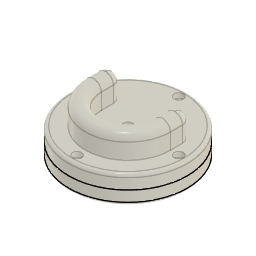
Spool Rod Holder (Autodesk Fusion 360 design; units mm, degrees)
Autodesk Fusion 360 part; units mm, degrees
sketch "Sketch1" plane through (0, 0, 0) normal (0, 0, 1) x (1, 0, 0) in component "Internal Rod Holder"
  circle A0 centre (0, 0) radius 16.875
  circle A1 centre (0, 0) radius 26.875
  line L0 (0, 16.875) -> (30, 16.875) construction
  line L1 (0, 16.875) -> (-30, 16.875) construction
  line L2 (-21.5932, 16) -> (-11.5932, 16)
  line L3 (-11.5932, 16) -> (-11.5932, 16.875)
  line L4 (-11.5932, 16.875) -> (-21.5932, 16.875)
  line L5 (-21.5932, 16.875) -> (-21.5932, 16)
  line L6 (5.3634, 16) -> (15.3634, 16)
  line L7 (15.3634, 16) -> (15.3634, 16.875)
  line L8 (15.3634, 16.875) -> (5.3634, 16.875)
  line L9 (5.3634, 16.875) -> (5.3634, 16)
  circle A2 centre (0, 0) radius 37.5
  line L10 (-33.9153, 16) -> (33.9153, 16)
  line L11 (-33.9153, 16) -> (-21.5932, 16)
  line L12 (15.3634, 16) -> (33.9153, 16)
  line L13 (0.0001, -26.875) -> (0.0001, -37.5)
  line L14 (0.0001, 26.875) -> (0.0001, 37.5)
  line L15 (-26.875, 0) -> (-37.5, 0)
  line L16 (26.875, 0) -> (37.5, 0)
  point P0 (-32, 16)
  point P1 (0.0001, 32.1875)
  point P2 (24.6393, 16)
  point P3 (-32.1875, 0)
  point P4 (32.1875, 0)
  point P5 (0.0001, -32.1875)
  dimension "d2" = 33.75
  dimension "d3" = 53.75
  dimension "d4" = 10
  dimension "d5" = 10
  dimension "d6" = 75
  dimension "d28" = 10.625
  constraint coincident A0.centre A1.centre
  constraint concentric A0 A1
  constraint coincident A0 L0.start
  constraint tangent A0 L0
  constraint horizontal L0
  constraint tangent A0 L1
  constraint horizontal L2
  constraint vertical L3
  constraint horizontal L4
  constraint vertical L5
  constraint coincident A1 L2.start
  constraint horizontal L6
  constraint vertical L7
  constraint horizontal L8
  constraint vertical L9
  constraint coincident A0 L6.start
  constraint concentric A1 A2
  constraint coincident A2 L10.start
  constraint coincident A2 L10.end
  constraint parallel L6 L10
  constraint coincident L10 P0
  constraint perpendicular L5 L11
  constraint perpendicular L7 L12
  constraint coincident A1 L13.start
  constraint coincident A2 L13.end
  constraint perpendicular L0 L13
  constraint coincident A1 L14.start
  constraint coincident A2 L14.end
  constraint parallel L13 L14
  constraint midpoint L14 P1
  constraint midpoint L12 P2
  constraint coincident A1 L15.start
  constraint coincident A2 L15.end
  constraint horizontal L15
  constraint coincident A1 L16.start
  constraint coincident A2 L16.end
  constraint parallel L15 L16
  constraint midpoint L15 P3
  constraint midpoint L16 P4
  constraint horizontal P3 P4
  constraint midpoint L13 P5
  measures "d2" diameter of A0
  measures "d3" diameter of A1
  measures "d4" distance of L2.start L2.end
  measures "d5" distance of L6.start L6.end
  measures "d6" diameter of A2
  measures "d28" distance of A1 A2
cylinder "CylinderPrimitive1" add diameter 75 height 8.75 placed x (1, 0, 0) y (0, 1, 0) z (0, 0, 1) at (0, 0, 0) makes body 1 in component "Internal Rod Holder"
cylinder "CylinderPrimitive2" add diameter 53.75 height 15 placed x (1, 0, 0) y (0, 1, 0) z (0, 0, 1) at (0, 0, 8.75) bodies 1 in component "Internal Rod Holder"
box "BoxPrimitive1" cut length 27.0154 width 53.75 height -15 placed x (0, 1, 0) y (-1, 0, 0) z (0, 0, 1) at (26.875, 0, 23.75) bodies 1 in component "Internal Rod Holder"
cylinder "CylinderPrimitive3" cut diameter 33.75 height 15 placed x (1, 0, 0) y (0, 1, 0) z (0, 0, 1) at (0, 0, 8.75) bodies 1 in component "Internal Rod Holder"
box "BoxPrimitive2" add length 12.656 width 10 height 15 placed x (0, 1, 0) y (-1, 0, 0) z (0, 0, 1) at (-16.875, 0, 8.75) bodies 1 in component "Internal Rod Holder"
box "BoxPrimitive3" add length 12.656 width 10 height 15 placed x (0, 1, 0) y (-1, 0, 0) z (0, 0, 1) at (26.875, 0, 8.75) bodies 1 in component "Internal Rod Holder"
sketch "Sketch8" plane through (0, 0, 8.75) normal (0, 0, 1) x (-1, 0, 0) in component "Internal Rod Holder"
  line L0 (-16.875, 0) -> (-16.875, -12.656)
  line L1 (-16.875, -12.656) -> (-26.875, -12.656)
  line L2 (-26.875, -12.656) -> (-26.875, 0)
  arc A0 (26.875, 0) -> (-26.875, 0) centre (0, 0) ccw
  line L3 (26.875, 0) -> (26.875, -12.656)
  line L4 (26.875, -12.656) -> (16.875, -12.656)
  line L5 (16.875, -12.656) -> (16.875, 0)
  arc A1 (16.875, 0) -> (-16.875, 0) centre (0, 0) ccw
  circle A2 centre (0, 0) radius 37.5
  point P0 (32.1875, 0)
  point P1 (32.1875, 0)
  point P2 (-0.0001, 32.1875)
  point P3 (-0.0001, 32.1875)
  point P4 (-32.1875, 0)
  point P5 (-32.1875, 0)
  point P6 (-0.0001, -32.1875)
  point P7 (-0.0001, -32.1875)
  constraint coincident P1 P0
  constraint coincident P3 P2
  constraint coincident P5 P4
  constraint coincident P7 P6
  constraint coincident A0.centre A1.centre
hole "Hole1" at (0.0001, -32.1875, 8.75) at (32.1875, 0, 8.75) at (0.0001, 32.1875, 8.75) at (0, 0, 8.75) at (-32.1875, 0, 8.75) direction (0, 0, -1) diameter 3.1 depth 25 tip angle 180 counterbore diameter 5.75 counterbore depth 3.2 bodies 1 in component "Internal Rod Holder"
cylinder "CylinderPrimitive4" add diameter 75 height -8.75 placed x (1, 0, 0) y (0, 1, 0) z (0, 0, 1) at (0, 0, 0) separate body makes body 2 in component "Internal Rod Holder"
copy_body "CutPasteBodies1" bodies 2 removing the originals makes body 3 in component "External Mount"
sketch "Sketch2" plane through (0, 0, -8.75) normal (0, 0, -1) x (1, 0, 0) in component "External Mount"
  circle A0 centre (0, 0) radius 37.5
  line L0 (-1.6558, 2.8773) -> (-3.3198, 0.0047)
  line L1 (-3.3198, 0.0047) -> (-1.6639, -2.8727)
  line L2 (-1.6639, -2.8727) -> (1.6558, -2.8773)
  line L3 (1.6558, -2.8773) -> (3.3198, -0.0047)
  line L4 (3.3198, -0.0047) -> (1.6639, 2.8727)
  line L5 (1.6639, 2.8727) -> (-1.6558, 2.8773)
  line L6 (1.66, 29.3125) -> (3.3199, 32.1875)
  line L7 (3.3199, 32.1875) -> (1.66, 35.0625)
  line L8 (1.66, 35.0625) -> (-1.6598, 35.0625)
  line L9 (-1.6598, 35.0625) -> (-3.3197, 32.1875)
  line L10 (-3.3197, 32.1875) -> (-1.6598, 29.3125)
  line L11 (-1.6598, 29.3125) -> (1.66, 29.3125)
  line L12 (-1.6598, -29.3125) -> (-3.3197, -32.1875)
  line L13 (-3.3197, -32.1875) -> (-1.6598, -35.0625)
  line L14 (-1.6598, -35.0625) -> (1.66, -35.0625)
  line L15 (1.66, -35.0625) -> (3.3199, -32.1875)
  line L16 (3.3199, -32.1875) -> (1.66, -29.3125)
  line L17 (1.66, -29.3125) -> (-1.6598, -29.3125)
  line L18 (-32.1876, -3.3198) -> (-29.3125, -1.66)
  line L19 (-29.3125, -1.66) -> (-29.3125, 1.6598)
  line L20 (-29.3125, 1.6598) -> (-32.1874, 3.3198)
  line L21 (-32.1874, 3.3198) -> (-35.0625, 1.66)
  line L22 (-35.0625, 1.66) -> (-35.0625, -1.6598)
  line L23 (-35.0625, -1.6598) -> (-32.1876, -3.3198)
  line L24 (32.1832, 3.3198) -> (29.3104, 1.6562)
  line L25 (29.3104, 1.6562) -> (29.3146, -1.6636)
  line L26 (29.3146, -1.6636) -> (32.1918, -3.3198)
  line L27 (32.1918, -3.3198) -> (35.0646, -1.6562)
  line L28 (35.0646, -1.6562) -> (35.0604, 1.6636)
  line L29 (35.0604, 1.6636) -> (32.1832, 3.3198)
  point P0 (32.1875, 0)
  point P1 (32.1875, 0)
  point P2 (-32.1875, 0)
  point P3 (-32.1875, 0)
  point P4 (0.0001, -32.1875)
  point P5 (0.0001, -32.1875)
  point P6 (0.0001, 32.1875)
  point P7 (0.0001, 32.1875)
  point P8 (0.0001, 32.1875)
  point P9 (0.0001, -32.1875)
  point P10 (-32.1875, 0)
  point P11 (32.1875, 0)
  dimension "d36" = 2.875
  dimension "d37" = 2.875
  dimension "d38" = 2.875
  dimension "d39" = 2.875
  dimension "d40" = 2.875
  constraint coincident P11 P1
  constraint coincident P10 P3
  constraint coincident A0.centre origin
  constraint coincident P9 P5
  constraint coincident P8 P7
  measures "d36" distance of A0.centre L5
  measures "d37" distance of P8 L11
  measures "d38" distance of P9 L17
  measures "d39" distance of P10 L23
  measures "d40" distance of P11 L29
extrude "Extrude1" cut sketch "Sketch2" against normal blind 3 contours L0 L1 L2 L3 L4 L5 | L6 L7 L8 L9 L10 L11 | L12 L13 L14 L15 L16 L17 | L18 L19 L20 L21 L22 L23 | L24 L25 L26 L27 L28 L29 bodies 3 in component "External Mount"
hole "Hole1'" at (-32.1875, 0, 0) at (0.0001, -32.1875, 0) at (0, 0, 0) at (32.1875, 0, 0) at (0.0001, 32.1875, 0) direction (0, 0, -1) diameter 3.1 depth 8.75 tip angle 180 bodies 3 in component "External Mount"
fillet "Fillet1" chord length 2.828 1 edges at (-13.5606, -34.9623, -8.75) on bodies 3 in component "External Mount"
fillet "Fillet1'" chord length 2.828 1 edges at (-34.9623, -13.5606, 8.75) on bodies 1 in component "Internal Rod Holder"
fillet "Fillet2" radius 5 12 edges at (-26.875, 6.328, 23.75) (0, -26.875, 23.75) (26.875, 6.328, 23.75) (21.875, 12.656, 23.75) (-21.875, 12.656, 23.75) (16.875, 6.328, 23.75) (0, -16.875, 23.75) (-16.875, 6.328, 23.75) (-26.875, 12.656, 16.25) (16.875, 12.656, 16.25) (26.875, 12.656, 16.25) (-16.875, 12.656, 16.25) on bodies 1 in component "Internal Rod Holder"
component "External Mount" placed x (1, 0, 0) y (0, 1, 0) z (0, 0, 1) at (0, 0, 0)
component "Internal Rod Holder" placed x (1, 0, 0) y (0, 1, 0) z (0, 0, 1) at (0, 0, 0)
